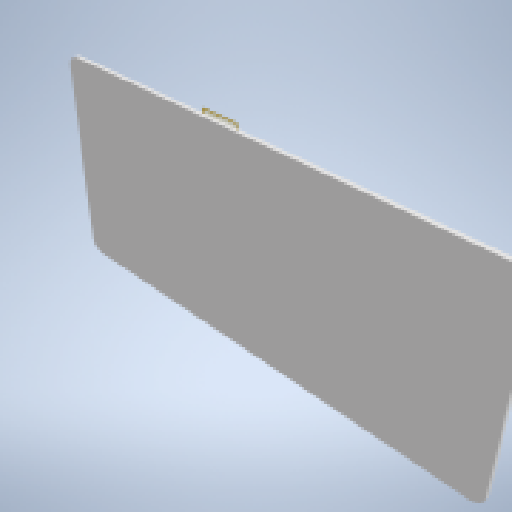
# Autodesk Inventor part: Part25
Saved by Autodesk Inventor 2023 (Build 270158000, 158)
## iProperties
Created: 2023-02-13
Part Number: Part25
Material: Generic
Document SubType Name: Modeling
Designer: klebe
Density: 1 g/cm^3
Appearance: Default
Author: klebe
Autodesk Inventor part; units mm, degrees
ref_plane "YZ Plane" through (0, 0, 0) normal (1, 0, 0) x (0, 1, 0)
ref_plane "XZ Plane" through (0, 0, 0) normal (0, 1, 0) x (-1, 0, 0)
ref_plane "XY Plane" through (0, 0, 0) normal (0, 0, 1) x (1, 0, 0)
ref_plane "Work Plane1" through (0, 0, 0) normal (0, 0, 1) x (1, 0, 0)
sketch "Sketch1" plane through (0, 0, 0) normal (0, 0, 1) x (1, 0, 0)
  line L0 (999.9981, -400) -> (999.9981, 400) projected
  ellipse E0 centre (949.9981, 400) end of major axis (949.9981, 450) minor radius 50 (999.9981, 400) -> (949.9981, 450) ccw projected
  ellipse E1 centre (949.9981, -400) end of major axis (949.9981, -350) minor radius 50 (949.9981, -450) -> (999.9981, -400) ccw projected
  arc A0 (-1000, -400) -> (-950, -450) centre (-950, -400) ccw projected
  line L1 (-1000, 400) -> (-1000, -400) projected
  arc A1 (-950, 450) -> (-1000, 400) centre (-950, 400) ccw projected
  line L2 (949.9981, 450) -> (-950, 450)
  line L3 (-950, -450) -> (949.9981, -450)
  point P0 (0, 0)
  constraints: 4 end point, 3 horizontal, 2 other
extrude "Extrusion1" add sketch "Sketch1" along normal blind 20
body "Solid1"
